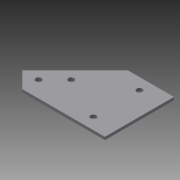
# Autodesk Inventor part: SideGusset
Saved by Autodesk Inventor 2013 (Build 170138000, 138)
## iProperties
Created: 2014-01-18
Part Number: SideGusset
Material: Generic
Document SubType Name: Modeling
Designer: 215152
Density: 1 g/cm^3
Author: 215152
Autodesk Inventor part; units mm, degrees
ref_plane "YZ Plane" through (0, 0, 0) normal (1, 0, 0) x (0, 1, 0)
ref_plane "XZ Plane" through (0, 0, 0) normal (0, 1, 0) x (-1, 0, 0)
ref_plane "XY Plane" through (0, 0, 0) normal (0, 0, 1) x (1, 0, 0)
sketch "Sketch1" plane through (0, 0, 0) normal (0, 1, 0) x (-1, 0, 0)
  line L0 (0, 0) -> (-50.8, 0)
  line L1 (0, 0) -> (50.8, 0) construction
  line L2 (-25.4, 0) -> (-25.4, 12.7)
  line L3 (-25.4, 0) -> (-12.7, 0) construction
  circle A0 centre (-25.4, 12.7) radius 3.175
  line L4 (-25.4, 12.7) -> (-25.4, 63.5)
  circle A1 centre (-25.4, 63.5) radius 3.175
  line L5 (-50.8, 0) -> (-50.8, 76.2)
  line L6 (-50.8, 0) -> (25.4, 0) construction
  line L7 (0, 0) -> (76.2, 76.2)
  line L8 (0, 0) -> (107.7631, 0) construction
  line L9 (76.2, 76.2) -> (-50.8, 76.2)
  line L10 (76.2, 76.2) -> (58.2395, 58.2395)
  line L11 (76.2, 76.2) -> (101.6, 76.2) construction
  line L12 (58.2395, 58.2395) -> (40.279, 76.2)
  line L13 (49.2592, 67.2197) -> (40.279, 58.2395)
  line L14 (49.2592, 67.2197) -> (61.9592, 67.2197) construction
  line L15 (40.279, 58.2395) -> (22.3185, 40.279)
  circle A2 centre (22.3185, 40.279) radius 3.175
  circle A3 centre (40.279, 58.2395) radius 3.175
  dimension "d0" = 50.8
  dimension "d1" = 180
  dimension "d2" = 12.7
  dimension "d3" = 90
  dimension "d4" = 6.35
  dimension "d5" = 50.8
  dimension "d6" = 6.35
  dimension "d7" = 76.2
  dimension "d8" = 90
  dimension "d9" = 45
  dimension "d10" = 25.4
  dimension "d11" = 135
  dimension "d12" = 12.7
  dimension "d13" = 135
  dimension "d14" = 25.4
  dimension "d15" = 180
  dimension "d16" = 6.35
  dimension "d17" = 6.35
  constraints: 32 end point, 7 horizontal, 6 equal length, 4 centre point, 4 coincident, 4 perpendicular, 2 collinear, 2 midpoint, 2 parallel, 1 point on line
  measures "d0" distance of L0.start L0.end
  measures "d1" angle of L0 L1
  measures "d2" distance of L2.start L2.end
  measures "d3" angle of L3 L2
  measures "d4" diameter of A0
  measures "d5" distance of L4.start L4.end
  measures "d6" diameter of A1
  measures "d7" distance of L0.end L5.end
  measures "d8" angle of L6 L5
  measures "d9" angle of L8 L7
  measures "d10" distance of L7.end L10.end
  measures "d11" angle of L10 L11
  measures "d12" distance of L13.start L13.end
  measures "d13" angle of L13 L14
  measures "d14" distance of L13.end L15.end
  measures "d15" angle of L15 L13
  measures "d16" diameter of A2
  measures "d17" diameter of A3
extrude "Extrusion1" add sketch "Sketch1" along normal blind 3.175 contours L0 L5 L9 L12 L7
body "Solid1"
